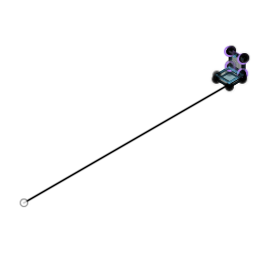
poop-bucket-bucket (Autodesk Fusion 360 design; units mm, degrees)
Autodesk Fusion 360 part; units mm, degrees
sketch "Sketch5" plane through (0, 0, 0) normal (0, 0, 1) x (1, 0, 0)
  line L0 (0, 0) -> (180, 0)
  line L1 (180, 0) -> (180, 80)
  line L2 (180, 80) -> (0, 80)
  line L3 (0, 80) -> (0, 0)
  line L4 (180, 0) -> (130, 0)
  line L5 (130, 0) -> (130, 40)
  line L6 (130, 40) -> (180, 40)
  line L7 (180, 40) -> (180, 0)
  dimension "d5" = 180
  dimension "d6" = 80
  dimension "d7" = 50
  dimension "d8" = 40
  constraint horizontal L0
  constraint vertical L1
  constraint horizontal L2
  constraint vertical L3
  constraint coincident L0.start L3.end
  constraint horizontal L4
  constraint vertical L5
  constraint horizontal L6
  constraint vertical L7
  measures "d5" distance of L0.start L0.end
  measures "d6" distance of L0.start L2.end
  measures "d7" distance of L0.end L4.end
  measures "d8" distance of L0.end L6.end
sketch "Sketch6" plane through (0, 0, 50) normal (0, 0, 1) x (-1, 0, 0)
  line L0 (-130, -40) -> (-180, -40)
  line L1 (-180, -40) -> (-180, -80)
  line L2 (-180, -80) -> (0, -80)
  line L3 (0, -80) -> (0, 0)
  line L4 (0, 0) -> (-130, 0)
  line L5 (-130, 0) -> (-130, -40)
  line L6 (-4, -76) -> (-126, -76)
  line L7 (-126, -76) -> (-126, -4)
  line L8 (-126, -4) -> (-4, -4)
  line L9 (-4, -4) -> (-4, -76)
  line L10 (-126, -76) -> (-176, -76)
  line L11 (-176, -76) -> (-176, -44)
  line L12 (-176, -44) -> (-126, -44)
  line L13 (-126, -44) -> (-126, -76)
  dimension "d11" = 4
  dimension "d12" = 4
  dimension "d13" = 4
  dimension "d14" = 4
  dimension "d15" = 4
  dimension "d16" = 4
  constraint horizontal L6
  constraint vertical L7
  constraint horizontal L8
  constraint vertical L9
  constraint horizontal L10
  constraint vertical L11
  constraint horizontal L12
  constraint vertical L13
  measures "d11" distance of L4 L8
  measures "d12" distance of L3 L9
  measures "d13" distance of L2 L6
  measures "d14" distance of L5 L7
  measures "d15" distance of L0 L12
  measures "d16" distance of L1 L11
sketch "Sketch7" plane through (0, 0, 50) normal (0, 0, 1) x (-1, 0, 0)
  line L0 (-4, -76) -> (-176, -76)
  line L1 (-176, -76) -> (-176, -44)
  line L2 (-176, -44) -> (-126, -44)
  line L3 (-126, -44) -> (-126, -4)
  line L4 (-126, -4) -> (-4, -4)
  line L5 (-4, -4) -> (-4, -76)
  line L6 (-130, -40) -> (-180, -40)
  line L7 (-180, -40) -> (-180, -80)
  line L8 (-180, -80) -> (0, -80)
  line L9 (0, -80) -> (0, 0)
  line L10 (0, 0) -> (-130, 0)
  line L11 (-130, 0) -> (-130, -40)
  line L12 (-4, -76) -> (0, -76)
  line L13 (-176, -44) -> (-176, -40)
  constraint coincident L0.start L5.end
  constraint coincident L9 L12.end
  constraint perpendicular L9 L12
  constraint coincident L1.end L2.start
  constraint coincident L6 L13.end
  constraint perpendicular L6 L13
sketch "Sketch8" plane through (0, 40, 0) normal (0, -1, 0) x (1, 0, 0)
  line L0 (180, 50) -> (180, 110)
  line L1 (180, 110) -> (176, 110)
  line L2 (176, 110) -> (176, 50)
  line L3 (176, 50) -> (180, 50)
  line L4 (176, 50) -> (180, 50)
  constraint coincident L2.end L3.start
  constraint coincident L0 L3.end
  constraint perpendicular L0 L3
sketch "Sketch9" plane through (0, 0, 110) normal (0, 0, 1) x (-1, 0, 0)
  line L0 (-180, -40) -> (-180, -80)
  line L1 (-180, -80) -> (0, -80)
  line L2 (0, -76) -> (-176, -76)
  line L3 (-176, -76) -> (-176, -40)
  line L4 (0, -80) -> (0, -76)
  line L5 (-176, -40) -> (-180, -40)
  line L6 (0, -80) -> (0, -76)
  constraint coincident L1.end L4.start
  constraint coincident L2 L4.end
  constraint perpendicular L2 L4
sketch "Sketch10" plane through (0, 80, 0) normal (0, 1, 0) x (-1, 0, 0)
  spline S0 degree 3 poles (-63.037188, 47.973181) (-57.805899, 55.776696) (-62.188829, 66.234353) (-72.120703, 68.166657) knots 0 0 0 0 1 1 1 1
  spline S1 degree 3 poles (-72.120703, 68.166657) (-66.968789, 73.015993) (-71.009453, 80.172126) (-76.645078, 82.707205) knots 0 0 0 0 1 1 1 1
  spline S2 degree 3 poles (-76.645078, 82.707205) (-79.507501, 83.994509) (-80.596523, 85.515174) (-81.546485, 87.100136) knots 0 0 0 0 1 1 1 1
  spline S3 degree 3 poles (-81.546485, 87.100136) (-83.367188, 90.128768) (-84.036953, 94.472168) (-88.819297, 96.945176) knots 0 0 0 0 1 1 1 1
  spline S4 degree 3 poles (-88.819297, 96.945176) (-92.113359, 98.651738) (-96.771718, 99.105604) (-99.272031, 97.627324) knots 0 0 0 0 1 1 1 1
  spline S5 degree 3 poles (-99.272031, 97.627324) (-100.953827, 96.635137) (-99.00406, 96.178731) (-97.565468, 95.015411) knots 0 0 0 0 1 1 1 1
  spline S6 degree 3 poles (-97.565468, 95.015411) (-95.179296, 93.083106) (-95.065156, 90.017326) (-97.153672, 87.554161) knots 0 0 0 0 1 1 1 1
  spline S7 degree 3 poles (-97.153672, 87.554161) (-99.8375, 84.381701) (-101.995547, 83.617638) (-104.421406, 82.707365) knots 0 0 0 0 1 1 1 1
  spline S8 degree 3 poles (-104.421406, 82.707365) (-110.205939, 80.539475) (-114.189452, 73.016153) (-109.040078, 68.166817) knots 0 0 0 0 1 1 1 1
  spline S9 degree 3 poles (-109.040078, 68.166817) (-119.120703, 66.204827) (-123.416955, 55.456818) (-117.798632, 47.618536) knots 0 0 0 0 1 1 1 1
  spline S10 degree 3 poles (-117.798632, 47.618536) (-124.786015, 45.986422) (-130, 39.730723) (-130, 32.242164) knots 0 0 0 0 1 1 1 1
  spline S11 degree 3 poles (-130, 32.242164) (-130, 27.415211) (-127.82957, 23.101656) (-124.418985, 20.20193) knots 0 0 0 0 1 1 1 1
  line L0 (-124.418985, 20.20193) -> (-54.301016, 20.20193)
  spline S12 degree 3 poles (-54.301016, 20.20193) (-50.892813, 23.101661) (-48.72, 27.415056) (-48.72, 32.242164) knots 0 0 0 0 1 1 1 1
  spline S13 degree 3 poles (-48.72, 32.242164) (-48.72, 40.469859) (-55.005547, 47.221657) (-63.037188, 47.973181) knots 0 0 0 0 1 1 1 1
  line L1 (-180, 50) -> (0, 50)
  line L2 (0, 50) -> (0, 110)
  line L3 (0, 110) -> (-180, 110)
  line L4 (-180, 110) -> (-180, 50)
sketch "Sketch11" plane through (0, 78.1, 0) normal (0, 1, 0) x (-1, 0, 0)
  spline S0 degree 3 poles (-72.120703, 68.166657) (-63.027473, 66.397516) (-58.585649, 57.481991) (-61.915206, 50) knots -1 -1 -1 -1 -0.08443962 -0.08443962 -0.08443962 -0.08443962
  spline S1 degree 3 poles (-76.645078, 82.707205) (-71.009453, 80.172126) (-66.968789, 73.015993) (-72.120703, 68.166657) knots -1 -1 -1 -1 0 0 0 0
  spline S2 degree 3 poles (-81.546485, 87.100136) (-80.596523, 85.515174) (-79.507501, 83.994509) (-76.645078, 82.707205) knots -1 -1 -1 -1 0 0 0 0
  spline S3 degree 3 poles (-88.819297, 96.945176) (-84.036953, 94.472168) (-83.367188, 90.128768) (-81.546485, 87.100136) knots -1 -1 -1 -1 0 0 0 0
  spline S4 degree 3 poles (-99.272031, 97.627324) (-96.771718, 99.105604) (-92.113359, 98.651738) (-88.819297, 96.945176) knots -1 -1 -1 -1 0 0 0 0
  spline S5 degree 3 poles (-97.565468, 95.015411) (-99.00406, 96.178731) (-100.953827, 96.635137) (-99.272031, 97.627324) knots -1 -1 -1 -1 0 0 0 0
  spline S6 degree 3 poles (-97.153672, 87.554161) (-95.065156, 90.017326) (-95.179296, 93.083106) (-97.565468, 95.015411) knots -1 -1 -1 -1 0 0 0 0
  spline S7 degree 3 poles (-104.421406, 82.707365) (-101.995547, 83.617638) (-99.8375, 84.381701) (-97.153672, 87.554161) knots -1 -1 -1 -1 0 0 0 0
  spline S8 degree 3 poles (-109.040078, 68.166817) (-114.189452, 73.016153) (-110.205939, 80.539475) (-104.421406, 82.707365) knots -1 -1 -1 -1 0 0 0 0
  spline S9 degree 3 poles (-119.170519, 50) (-122.517702, 57.482369) (-118.131108, 66.397432) (-109.040078, 68.166817) knots -0.90183199 -0.90183199 -0.90183199 -0.90183199 0 0 0 0
  line L0 (-95.271606, 70.572289) -> (-74.970963, 70.04733) construction
  line L1 (-74.970963, 70.04733) -> (-74.728394, 79.427711) construction
  line L2 (-74.728394, 79.427711) -> (-95.029037, 79.95267) construction
  line L3 (-95.029037, 79.95267) -> (-95.271606, 70.572289) construction
  line L4 (-119.170519, 50) -> (-61.915206, 50)
  dimension "d43" = 10
sketch "Sketch12" plane through (0, 78.1, 0) normal (0, 1, 0) x (-1, 0, 0)
  line L0 (-95.287543, 69.956012) -> (-95.029389, 79.939051)
  line L1 (-95.029389, 79.939051) -> (-93.803641, 79.907354)
  line L2 (-93.803641, 79.907354) -> (-94.061795, 69.924315)
  line L3 (-94.061795, 69.924315) -> (-95.287543, 69.956012)
  spline S0 degree 3 poles (-72.120703, 68.166657) (-63.027473, 66.397516) (-58.585649, 57.481991) (-61.915206, 50) knots -1 -1 -1 -1 -0.08443962 -0.08443962 -0.08443962 -0.08443962
  spline S1 degree 3 poles (-76.645078, 82.707205) (-71.009453, 80.172126) (-66.968789, 73.015993) (-72.120703, 68.166657) knots -1 -1 -1 -1 0 0 0 0
  spline S2 degree 3 poles (-81.546485, 87.100136) (-80.596523, 85.515174) (-79.507501, 83.994509) (-76.645078, 82.707205) knots -1 -1 -1 -1 0 0 0 0
  spline S3 degree 3 poles (-88.819297, 96.945176) (-84.036953, 94.472168) (-83.367188, 90.128768) (-81.546485, 87.100136) knots -1 -1 -1 -1 0 0 0 0
  spline S4 degree 3 poles (-99.272031, 97.627324) (-96.771718, 99.105604) (-92.113359, 98.651738) (-88.819297, 96.945176) knots -1 -1 -1 -1 0 0 0 0
  spline S5 degree 3 poles (-97.565468, 95.015411) (-99.00406, 96.178731) (-100.953827, 96.635137) (-99.272031, 97.627324) knots -1 -1 -1 -1 0 0 0 0
  spline S6 degree 3 poles (-97.153672, 87.554161) (-95.065156, 90.017326) (-95.179296, 93.083106) (-97.565468, 95.015411) knots -1 -1 -1 -1 0 0 0 0
  spline S7 degree 3 poles (-104.421406, 82.707365) (-101.995547, 83.617638) (-99.8375, 84.381701) (-97.153672, 87.554161) knots -1 -1 -1 -1 0 0 0 0
  spline S8 degree 3 poles (-109.040078, 68.166817) (-114.189452, 73.016153) (-110.205939, 80.539475) (-104.421406, 82.707365) knots -1 -1 -1 -1 0 0 0 0
  spline S9 degree 3 poles (-119.170519, 50) (-122.517702, 57.482369) (-118.131108, 66.397432) (-109.040078, 68.166817) knots -0.90183199 -0.90183199 -0.90183199 -0.90183199 0 0 0 0
  line L4 (-87.151, 72.076086) -> (-85.888444, 71.886709)
  spline S10 degree 3 poles (-85.888444, 71.886709) (-86.013749, 71.544143) (-86.256236, 70.881215) (-86.786653, 70.416925) (-87.042978, 70.192555) knots 0 0 0 0 0.10747009 0.20797433 0.20797433 0.20797433 0.20797433
  spline S11 degree 3 poles (-87.042978, 70.192555) (-87.34739, 70.021715) (-87.993643, 69.659028) (-88.736198, 69.642145) (-89.128979, 69.633214) knots 0 0 0 0 0.10312117 0.21892194 0.21892194 0.21892194 0.21892194
  spline S12 degree 3 poles (-89.128979, 69.633214) (-89.621732, 69.678688) (-90.564027, 69.765647) (-91.278869, 70.381614) (-91.619899, 70.675474) knots 0 0 0 0 0.14436887 0.2760774 0.2760774 0.2760774 0.2760774
  spline S13 degree 3 poles (-91.619899, 70.675474) (-91.880847, 71.060122) (-92.4446, 71.891114) (-92.466685, 72.89904) (-92.478547, 73.44042) knots 0 0 0 0 0.13656936 0.29504448 0.29504448 0.29504448 0.29504448
  spline S14 degree 3 poles (-92.478547, 73.44042) (-92.438608, 73.998404) (-92.364473, 75.03413) (-91.749305, 75.865486) (-91.465551, 76.24896) knots 0 0 0 0 0.16381985 0.30408105 0.30408105 0.30408105 0.30408105
  spline S15 degree 3 poles (-91.465551, 76.24896) (-91.115766, 76.534017) (-90.399204, 77.11798) (-89.474783, 77.168101) (-89.001612, 77.193755) knots 0 0 0 0 0.13181373 0.2700304 0.2700304 0.2700304 0.2700304
  spline S16 degree 3 poles (-89.001612, 77.193755) (-88.544529, 77.144258) (-87.648774, 77.047256) (-86.983276, 76.441647) (-86.657366, 76.145067) knots 0 0 0 0 0.13410505 0.26280803 0.26280803 0.26280803 0.26280803
  spline S17 degree 3 poles (-86.657366, 76.145067) (-86.399569, 75.755215) (-85.840301, 74.909463) (-85.820549, 73.891605) (-85.809902, 73.342931) knots 0 0 0 0 0.13742972 0.29814259 0.29814259 0.29814259 0.29814259
  spline S18 degree 3 poles (-85.809902, 73.342931) (-85.811508, 73.297542) (-85.815363, 73.188589) (-85.821553, 73.079742) (-85.825164, 73.016241) knots 0 0 0 0 0.01362508 0.03270546 0.03270546 0.03270546 0.03270546
  line L5 (-85.825164, 73.016241) -> (-91.218456, 73.155707)
  spline S19 degree 3 poles (-91.218456, 73.155707) (-91.192425, 72.791673) (-91.144397, 72.120013) (-90.765174, 71.566695) (-90.591487, 71.313271) knots 0 0 0 0 0.10717868 0.19774945 0.19774945 0.19774945 0.19774945
  spline S20 degree 3 poles (-90.591487, 71.313271) (-90.380387, 71.12298) (-89.95425, 70.738849) (-89.383911, 70.673733) (-89.096108, 70.640875) knots 0 0 0 0 0.08305336 0.16765533 0.16765533 0.16765533 0.16765533
  spline S21 degree 3 poles (-89.096108, 70.640875) (-88.882219, 70.64798) (-88.46859, 70.661722) (-88.109509, 70.866388) (-87.936109, 70.965221) knots 0 0 0 0 0.06312425 0.12207286 0.12207286 0.12207286 0.12207286
  spline S22 degree 3 poles (-87.936109, 70.965221) (-87.778407, 71.106547) (-87.433022, 71.416068) (-87.250294, 71.843706) (-87.151, 72.076086) knots 0 0 0 0 0.06278045 0.13749631 0.13749631 0.13749631 0.13749631
  line L6 (-103.914159, 49.813108) -> (-85.96986, 50.017766) construction
  line L7 (-85.96986, 50.017766) -> (-86.085841, 60.186892) construction
  line L8 (-86.085841, 60.186892) -> (-104.03014, 59.982234) construction
  line L9 (-104.03014, 59.982234) -> (-103.914159, 49.813108) construction
  line L10 (-109.465848, 33.644768) -> (-81.410898, 33.591101) construction
  line L11 (-81.410898, 33.591101) -> (-81.399171, 39.721358) construction
  line L12 (-81.399171, 39.721358) -> (-109.454121, 39.775026) construction
  line L13 (-109.454121, 39.775026) -> (-109.465848, 33.644768) construction
  line L14 (-119.170519, 50) -> (-61.915206, 50)
  dimension "d46" = 10
  dimension "d47" = 10
sketch "Sketch13" plane through (0, 0, 0) normal (0, 0, -1) x (1, 0, 0)
  arc A0 (180, -50) -> (170, -40) centre (170, -50) ccw
  line L0 (170, -40) -> (135, -40)
  arc A1 (130, -35) -> (135, -40) centre (135, -35) ccw
  line L1 (130, -35) -> (130, -10)
  arc A2 (130, -10) -> (120, 0) centre (120, -10) ccw
  line L2 (120, 0) -> (10, 0)
  arc A3 (10, 0) -> (0, -10) centre (10, -10) ccw
  line L3 (0, -10) -> (0, -70)
  arc A4 (0, -70) -> (10, -80) centre (10, -70) ccw
  line L4 (10, -80) -> (170, -80)
  arc A5 (170, -80) -> (180, -70) centre (170, -70) ccw
  line L5 (180, -70) -> (180, -50)
  circle A6 centre (12, -2) radius 1.25
  circle A7 centre (12, -78) radius 1.25
  circle A8 centre (168, -78) radius 1.25
  dimension "d50" = 2.5
  dimension "d51" = 12
  dimension "d52" = 2
  dimension "d53" = 2.5
  dimension "d54" = 2
  dimension "d55" = 12
  dimension "d56" = 2.5
  dimension "d57" = 12
  dimension "d58" = 2
  measures "d50" diameter of A6
  measures "d51" distance of L3 A6.centre
  measures "d52" distance of L2 A6.centre
  measures "d53" diameter of A7
  measures "d54" distance of L4 A7.centre
  measures "d55" distance of L3 A7.centre
  measures "d56" diameter of A8
  measures "d57" distance of L5 A8.centre
  measures "d58" distance of L4 A8.centre
sketch "Sketch14" plane through (0, 0, 0) normal (0, -1, 0) x (1, 0, 0)
  line L0 (120, 47) -> (10, 47)
  line L1 (10, 47) -> (10, 0)
  line L2 (10, 0) -> (120, 0)
  line L3 (120, 0) -> (120, 47)
  line L4 (0, 25) -> (176, 25)
  line L5 (176, 25) -> (176, 56.725104)
  line L6 (176, 56.725104) -> (0, 56.725104)
  line L7 (0, 56.725104) -> (0, 25)
  dimension "d65" = 176
  constraint horizontal L4
  constraint vertical L5
  constraint horizontal L6
  constraint vertical L7
  measures "d65" distance of L4.start L4.end
sketch "Sketch15" plane through (0, 40, 0) normal (0, -1, 0) x (1, 0, 0)
  line L0 (176.000003, 25) -> (135.000002, 0)
  line L1 (135.000002, 0) -> (176.000003, 0)
  line L2 (176.000003, 0) -> (176.000003, 25)
  constraint horizontal L1
  constraint perpendicular L1 L2
sketch "Sketch16" plane through (0, 0, 4) normal (0, 0, 1) x (-1, 0, 0)
  arc A0 (-171, -44) -> (-176, -49) centre (-171, -49) ccw
  line L0 (-176, -49) -> (-176, -76)
  line L1 (-176, -76) -> (-9, -76)
  arc A1 (-9, -76) -> (-4, -71) centre (-9, -71) ccw
  line L2 (-4, -71) -> (-4, -9)
  arc A2 (-4, -9) -> (-9, -4) centre (-9, -9) ccw
  line L3 (-9, -4) -> (-121, -4)
  arc A3 (-121, -4) -> (-126, -9) centre (-121, -9) ccw
  line L4 (-126, -9) -> (-126, -39)
  arc A4 (-131, -44) -> (-126, -39) centre (-131, -39) ccw
  line L5 (-131, -44) -> (-171, -44)
  line L6 (-141.561257, -76.000004) -> (-141.561257, -44)
  constraint perpendicular L5 L6
sketch "Sketch17" plane through (0, 0, 4) normal (0, 0, 1) x (-1, 0, 0)
  arc A0 (-171, -44) -> (-176, -49) centre (-171, -49) ccw
  line L0 (-176, -49) -> (-176, -76)
  line L1 (-176, -76) -> (-9, -76)
  arc A1 (-9, -76) -> (-4, -71) centre (-9, -71) ccw
  line L2 (-4, -71) -> (-4, -9)
  arc A2 (-4, -9) -> (-9, -4) centre (-9, -9) ccw
  line L3 (-9, -4) -> (-121, -4)
  arc A3 (-121, -4) -> (-126, -9) centre (-121, -9) ccw
  line L4 (-126, -9) -> (-126, -39)
  arc A4 (-131, -44) -> (-126, -39) centre (-131, -39) ccw
  line L5 (-131, -44) -> (-171, -44)
sketch "Sketch18" plane through (0, 0, 0) normal (0, 0, 1) x (1, 0, 0)
  line L0 (250, 0) -> (430, 0)
  line L1 (430, 0) -> (430, 180)
  line L2 (430, 180) -> (250, 180)
  line L3 (250, 180) -> (250, 0)
  dimension "d76" = 180
  dimension "d77" = 180
  constraint horizontal L0
  constraint vertical L1
  constraint horizontal L2
  constraint vertical L3
  measures "d76" distance of L0.start L0.end
  measures "d77" distance of L0.start L2.end
extrude "Extrude12" add sketch "Sketch18" along normal blind 4 makes body 1
sketch "Sketch19" plane through (0, 0, 4) normal (0, 0, 1) x (-1, 0, 0)
  line L0 (-250, -180) -> (-250, 0)
  line L1 (-250, 0) -> (-430, 0)
  line L2 (-430, 0) -> (-430, -180)
  line L3 (-430, -180) -> (-250, -180)
  line L4 (-258, -8) -> (-422, -8)
  line L5 (-422, -8) -> (-422, -172)
  line L6 (-422, -172) -> (-258, -172)
  line L7 (-258, -172) -> (-258, -8)
  dimension "d80" = 164
  dimension "d81" = 164
  dimension "d82" = 8
  dimension "d83" = 8
  constraint horizontal L4
  constraint vertical L5
  constraint horizontal L6
  constraint vertical L7
  measures "d80" distance of L4.start L4.end
  measures "d81" distance of L4.start L6.end
  measures "d82" distance of L1 L4
  measures "d83" distance of L0 L7
extrude "Extrude13" add sketch "Sketch19" along normal blind 2 bodies 1
sketch "Sketch20" plane through (0, 0, 6) normal (0, 0, 1) x (-1, 0, 0)
  line L0 (-258, -8) -> (-258, -172)
  line L1 (-258, -172) -> (-422, -172)
  line L2 (-422, -172) -> (-422, -8)
  line L3 (-422, -8) -> (-258, -8)
  line L4 (-430, -180) -> (-250, -180)
  line L5 (-250, -180) -> (-250, 0)
  line L6 (-250, 0) -> (-430, 0)
  line L7 (-430, 0) -> (-430, -180)
  line L8 (-256, -174) -> (-424, -174)
  line L9 (-424, -174) -> (-424, -6)
  line L10 (-424, -6) -> (-256, -6)
  line L11 (-256, -6) -> (-256, -174)
  dimension "d86" = 168
  dimension "d87" = 168
  dimension "d88" = 6
  dimension "d89" = 6
  constraint horizontal L8
  constraint vertical L9
  constraint horizontal L10
  constraint vertical L11
  measures "d86" distance of L8.start L8.end
  measures "d87" distance of L8.start L10.end
  measures "d88" distance of L4 L8
  measures "d89" distance of L5 L11
extrude "Extrude14" add sketch "Sketch20" along normal blind 50 contours L8 L9 L10 L11 picked at (-367.333333, -6.666667) bodies 1
sketch "Sketch21" plane through (0, 0, 6) normal (0, 0, 1) x (-1, 0, 0)
  line L0 (-256, -6) -> (-256, -174)
  line L1 (-256, -174) -> (-424, -174)
  line L2 (-424, -174) -> (-424, -6)
  line L3 (-424, -6) -> (-256, -6)
  line L4 (-430, -180) -> (-250, -180)
  line L5 (-250, -180) -> (-250, 0)
  line L6 (-250, 0) -> (-430, 0)
  line L7 (-430, 0) -> (-430, -180)
  line L8 (-250, 0) -> (-256, 0)
  line L9 (-256, 0) -> (-256, -6)
  line L10 (-256, -6) -> (-250, -6)
  line L11 (-250, -6) -> (-250, 0)
  line L12 (-424, -6) -> (-430, -6)
  line L13 (-430, -6) -> (-430, 0)
  line L14 (-430, 0) -> (-424, 0)
  line L15 (-424, 0) -> (-424, -6)
  line L16 (-424, -174) -> (-430, -174)
  line L17 (-430, -174) -> (-430, -180)
  line L18 (-430, -180) -> (-424, -180)
  line L19 (-424, -180) -> (-424, -174)
  line L20 (-250, -180) -> (-256, -180)
  line L21 (-256, -180) -> (-256, -174)
  line L22 (-256, -174) -> (-250, -174)
  line L23 (-250, -174) -> (-250, -180)
  constraint horizontal L8
  constraint vertical L9
  constraint horizontal L10
  constraint vertical L11
  constraint coincident L0.start L3.end
  constraint coincident L5.end L6.start
  constraint horizontal L12
  constraint vertical L13
  constraint horizontal L14
  constraint vertical L15
  constraint coincident L6.end L7.start
  constraint coincident L2.end L3.start
  constraint horizontal L16
  constraint vertical L17
  constraint horizontal L18
  constraint vertical L19
  constraint coincident L4.start L7.end
  constraint coincident L1.end L2.start
  constraint horizontal L20
  constraint vertical L21
  constraint horizontal L22
  constraint vertical L23
  constraint coincident L0.end L1.start
  constraint coincident L4.end L5.start
extrude "Extrude15" add sketch "Sketch21" along normal blind 50 separate body contours L4 L5 L20 L21 L22 L23 picked at (-254, -176) makes body 2
extrude "Extrude16" add sketch "Sketch21" along normal blind 50 separate body contours L5 L6 L8 L9 L10 L11 picked at (-254, -4) makes body 3
extrude "Extrude17" add sketch "Sketch21" along normal blind 50 separate body contours L6 L7 L12 L13 L14 L15 picked at (-426, -4) makes body 4
extrude "Extrude18" add sketch "Sketch21" along normal blind 50 separate body contours L4 L7 L16 L17 L18 L19 picked at (-428, -178) makes body 5
sketch "Sketch22" plane through (0, 0, 56) normal (0, 0, 1) x (-1, 0, 0)
  line L0 (-250, -6) -> (-250, 0)
  line L1 (-250, 0) -> (-256, 0)
  line L2 (-256, 0) -> (-256, -6)
  line L3 (-256, -6) -> (-250, -6)
  line L4 (-250, -180) -> (-430, -180)
  line L5 (-430, -180) -> (-430, 0)
  line L6 (-430, 0) -> (-250, 0)
  line L7 (-250, 0) -> (-250, -180)
  line L8 (-256, -6) -> (-424.000006, -6)
  line L9 (-424.000006, -6) -> (-424.000006, -174.000003)
  line L10 (-424.000006, -174.000003) -> (-256, -174.000003)
  line L11 (-256, -174.000003) -> (-256, -6)
  constraint horizontal L4
  constraint vertical L5
  constraint horizontal L6
  constraint vertical L7
  constraint horizontal L8
  constraint vertical L9
  constraint horizontal L10
  constraint vertical L11
  constraint coincident L2.end L3.start
extrude "Extrude19" add sketch "Sketch22" along normal blind 6 separate body contours L2 L3 L4 L5 L6 L7 picked at (-312, -178.000001) makes body 6
extrude "Extrude20" add 1 faces at (254, 4, 56) along direction (0, 0, 1) blind 6 on bodies 3 bodies 1 2 4 5 3 6
sketch "Sketch23" plane through (0, 0, 62) normal (0, 0, 1) x (-1, 0, 0)
  line L0 (-256, -6) -> (-256, -174.000003)
  line L1 (-256, -174.000003) -> (-424.000006, -174.000003)
  line L2 (-424.000006, -174.000003) -> (-424.000006, -6)
  line L3 (-424.000006, -6) -> (-256, -6)
  line L4 (-250, -180) -> (-250, 0)
  line L5 (-250, 0) -> (-430, 0)
  line L6 (-430, 0) -> (-430, -180)
  line L7 (-430, -180) -> (-250, -180)
  line L8 (-250, -180) -> (-430, -180)
  line L9 (-430, -180) -> (-430, -186)
  line L10 (-430, -186) -> (-250, -186)
  line L11 (-250, -186) -> (-250, -180)
  line L12 (-250, -180) -> (-256, -180)
  line L13 (-256, -180) -> (-256, -210)
  line L14 (-256, -210) -> (-250, -210)
  line L15 (-250, -210) -> (-250, -180)
  line L16 (-250, -210) -> (-430, -210)
  line L17 (-430, -210) -> (-430, -204)
  line L18 (-430, -204) -> (-250, -204)
  line L19 (-250, -204) -> (-250, -210)
  line L20 (-430, -210) -> (-424, -210)
  line L21 (-424, -210) -> (-424, -180)
  line L22 (-424, -180) -> (-430, -180)
  line L23 (-430, -180) -> (-430, -210)
  dimension "d104" = 180
  dimension "d105" = 6
  dimension "d106" = 6
  dimension "d107" = 30
  dimension "d108" = 180
  dimension "d109" = 6
  dimension "d110" = 6
  dimension "d111" = 30
  constraint horizontal L8
  constraint vertical L9
  constraint horizontal L10
  constraint vertical L11
  constraint coincident L4.start L7.end
  constraint horizontal L12
  constraint vertical L13
  constraint horizontal L14
  constraint vertical L15
  constraint horizontal L16
  constraint vertical L17
  constraint horizontal L18
  constraint vertical L19
  constraint horizontal L20
  constraint vertical L21
  constraint horizontal L22
  constraint vertical L23
  measures "d104" distance of L4.start L6.end
  measures "d105" distance of L4.start L10.end
  measures "d106" distance of L4.start L12.end
  measures "d107" distance of L4.start L14.end
  measures "d108" distance of L14.end L16.end
  measures "d109" distance of L14.end L18.end
  measures "d110" distance of L16.end L20.end
  measures "d111" distance of L16.end L6.end
extrude "Extrude21" add sketch "Sketch23" along normal blind 6 separate body contours L7 L8 L10 L11 L12 L13 L15 | L7 L8 L10 L13 L21 | L10 L13 L15 L18 | L7 L8 L9 L10 L21 L22 L23 | L10 L13 L18 L21 | L13 L14 L15 L16 L18 L19 | L10 L18 L21 L23 | L13 L16 L18 L21 | L16 L17 L18 L20 L21 L23 picked at (-254, -184) picked at (-368, -182) picked at (-254, -192) picked at (-428, -184) picked at (-368, -198) picked at (-254, -208) picked at (-428, -192) picked at (-368, -206) picked at (-428, -208) makes body 7
extrude "Extrude22" add sketch "Sketch23" along normal blind 180 separate body contours L10 L13 L18 L21 picked at (-368, -198) makes body 8
extrude "Extrude23" add sketch "Sketch23" along normal blind 180 separate body contours L7 L8 L10 L11 L12 L13 L15 | L7 L8 L9 L10 L21 L22 L23 | L13 L14 L15 L16 L18 L19 | L16 L17 L18 L20 L21 L23 picked at (-254, -184) picked at (-428, -184) picked at (-254, -208) picked at (-428, -208) makes body 9 at (424, 184, 122) makes body 10 at (250, 208, 122) makes body 11 at (424, 208, 122) makes body 12 at (250, 184, 122)
extrude "Extrude24" cut 1 faces at (368, 198, 242) along direction (0, 0, -1) blind 6 on bodies 8 bodies 8
extrude "Extrude25" cut sketch "Sketch23" along normal blind 6 contours L10 L13 L18 L21 picked at (-368, -198) bodies 8
sketch "Sketch24" plane through (256, 0, 0) normal (1, 0, 0) x (0, 1, 0)
  line L0 (204, 62) -> (210, 62)
  line L1 (210, 62) -> (210, 242)
  line L2 (210, 242) -> (204, 242)
  line L3 (204, 242) -> (204, 62)
  line L4 (186.000003, 68.000001) -> (180.000003, 68.000001)
  line L5 (180.000003, 68.000001) -> (180.000003, 62.000001)
  line L6 (180.000003, 62.000001) -> (186.000003, 62.000001)
  line L7 (186.000003, 62.000001) -> (186.000003, 68.000001)
  line L8 (204, 62) -> (210.000003, 62)
  line L9 (210.000003, 62) -> (210.000003, 68.000001)
  line L10 (210.000003, 68.000001) -> (204, 68.000001)
  line L11 (204, 68.000001) -> (204, 62)
  constraint horizontal L4
  constraint vertical L5
  constraint horizontal L6
  constraint vertical L7
  constraint horizontal L8
  constraint vertical L9
  constraint horizontal L10
  constraint vertical L11
  constraint coincident L0.start L3.end
extrude "Extrude26" add sketch "Sketch24" along normal blind 168 contours L0 L1 L3 L8 L9 L10 L11 picked at (206, 66.000001) bodies 8 9 12 10 11
extrude "Extrude27" add sketch "Sketch24" along normal blind 168 contours L4 L5 L6 L7 picked at (182.000003, 66.000001) bodies 1 2 4 5 9 8 12
sketch "Sketch25" plane through (0, 186, 0) normal (0, 1, 0) x (-1, 0, 0)
  line L0 (-256, 62) -> (-250, 62)
  line L1 (-250, 62) -> (-250, 242)
  line L2 (-250, 242) -> (-256, 242)
  line L3 (-256, 242) -> (-256, 236)
  line L4 (-256, 236) -> (-256, 68)
  line L5 (-256, 68) -> (-424, 68)
  line L6 (-424, 68) -> (-424, 236)
  line L7 (-424, 236) -> (-424, 242)
  line L8 (-424, 242) -> (-430, 242)
  line L9 (-430, 242) -> (-430, 62)
  line L10 (-430, 62) -> (-424, 62)
  line L11 (-424, 62) -> (-256, 62)
  line L12 (-256, 62) -> (-250.000004, 62)
  line L13 (-250.000004, 62) -> (-250.000004, 68.000001)
  line L14 (-250.000004, 68.000001) -> (-256, 68.000001)
  line L15 (-256, 68.000001) -> (-256, 62)
  line L16 (-430, 62) -> (-424, 62)
  line L17 (-424, 62) -> (-424, 68)
  line L18 (-424, 68) -> (-430, 68)
  line L19 (-430, 68) -> (-430, 62)
  constraint horizontal L12
  constraint vertical L13
  constraint horizontal L14
  constraint vertical L15
  constraint coincident L0.start L11.end
  constraint horizontal L16
  constraint vertical L17
  constraint horizontal L18
  constraint vertical L19
  constraint coincident L5.end L6.start
  constraint coincident L9.end L10.start
extrude "Extrude28" add sketch "Sketch25" along normal blind 18 separate body contours L9 L10 L16 L17 L18 L19 picked at (-426, 64) makes body 13
extrude "Extrude29" add sketch "Sketch25" along normal blind 18 separate body contours L0 L1 L12 L13 L14 L15 picked at (-254, 64) makes body 14
sketch "Sketch26" plane through (424, 0, 0) normal (-1, 0, 0) x (0, -1, 0)
  line L0 (-210.000003, 68.000001) -> (-204, 68)
  line L1 (-204, 68) -> (-204, 236)
  line L2 (-204, 236) -> (-204, 242)
  line L3 (-204, 242) -> (-210, 242)
  line L4 (-210, 242) -> (-210.000003, 68.000001)
  line L5 (-210, 242) -> (-204, 242)
  line L6 (-204, 242) -> (-204, 236)
  line L7 (-204, 236) -> (-210, 236)
  line L8 (-210, 236) -> (-210, 242)
  line L9 (-186.000003, 242.000004) -> (-180.000003, 242.000004)
  line L10 (-180.000003, 242.000004) -> (-180.000003, 236.000004)
  line L11 (-180.000003, 236.000004) -> (-186.000003, 236.000004)
  line L12 (-186.000003, 236.000004) -> (-186.000003, 242.000004)
  constraint horizontal L5
  constraint vertical L6
  constraint horizontal L7
  constraint vertical L8
  constraint coincident L1.end L2.start
  constraint coincident L3.end L4.start
  constraint horizontal L9
  constraint vertical L10
  constraint horizontal L11
  constraint vertical L12
sketch "Sketch27" plane through (0, 204, 0) normal (0, -1, 0) x (1, 0, 0)
  line L0 (250, 62) -> (430, 62)
  line L1 (430, 62) -> (430, 242)
  line L2 (430, 242) -> (424, 242)
  line L3 (424, 242) -> (424, 236)
  line L4 (424, 236) -> (424, 68)
  line L5 (424, 68) -> (256, 68)
  line L6 (256, 68) -> (256, 236)
  line L7 (256, 236) -> (256, 242)
  line L8 (256, 242) -> (250, 242)
  line L9 (250, 242) -> (250, 62)
  line L10 (250, 242) -> (256, 242)
  line L11 (256, 242) -> (256, 236)
  line L12 (256, 236) -> (250, 236)
  line L13 (250, 236) -> (250, 242)
  line L14 (424, 242) -> (430, 242)
  line L15 (430, 242) -> (430, 236)
  line L16 (430, 236) -> (424, 236)
  line L17 (424, 236) -> (424, 242)
  constraint horizontal L10
  constraint vertical L11
  constraint horizontal L12
  constraint vertical L13
  constraint coincident L6.end L7.start
  constraint coincident L8.end L9.start
  constraint horizontal L14
  constraint vertical L15
  constraint horizontal L16
  constraint vertical L17
  constraint coincident L1 L15.end
  constraint coincident L2.end L3.start
extrude "Extrude30" add sketch "Sketch26" along normal blind 168 separate body contours L2 L3 L4 L5 L6 L7 L8 picked at (-208, 238) makes body 15
extrude "Extrude31" add sketch "Sketch26" along normal blind 168 separate body contours L9 L10 L11 L12 picked at (-184.000003, 240.000004) makes body 16
extrude "Extrude32" add sketch "Sketch27" along normal blind 18 separate body contours L1 L2 L3 L14 L15 L16 L17 picked at (428, 238) makes body 17
extrude "Extrude33" add sketch "Sketch27" along normal blind 18 separate body contours L7 L8 L9 L10 L11 L12 L13 picked at (252, 238) makes body 18
sketch "Sketch28" plane through (0, 0, 242.000004) normal (0, 0, 1) x (-1, 0, 0)
  line L0 (-424, -180.000003) -> (-424, -186.000003)
  line L1 (-424, -186.000003) -> (-256, -186.000003)
  line L2 (-256, -186.000003) -> (-256, -180.000003)
  line L3 (-256, -180.000003) -> (-424, -180.000003)
  line L4 (-330, -190) -> (-350, -190)
  line L5 (-350, -190) -> (-350, -155)
  line L6 (-350, -155) -> (-330, -155)
  line L7 (-330, -155) -> (-330, -190)
  line L8 (-335, -185) -> (-345, -185)
  line L9 (-345, -185) -> (-345, -160)
  line L10 (-345, -160) -> (-335, -160)
  line L11 (-335, -160) -> (-335, -185)
  line L12 (-250, -210) -> (-250, -180)
  line L13 (-430, -180) -> (-430, -210)
  line L14 (-250, -210) -> (-430, -210)
  dimension "d138" = 80
  dimension "d139" = 85
  dimension "d140" = 80
  dimension "d141" = 20
  dimension "d142" = 25
  constraint horizontal L4
  constraint vertical L5
  constraint horizontal L6
  constraint vertical L7
  constraint horizontal L8
  constraint vertical L9
  constraint horizontal L10
  constraint vertical L11
  measures "d138" distance of L7 L12
  measures "d139" distance of L9 L13
  measures "d140" distance of L5 L13
  measures "d141" distance of L4 L14
  measures "d142" distance of L8 L14
extrude "Extrude34" add sketch "Sketch28" along normal blind 10 contours L3 L5 L6 L7 L9 L10 L11 | L1 L3 L5 L7 L8 L9 L11 | L1 L4 L5 L7 picked at (-348.333333, -165.000001) picked at (-348.333333, -183.666668) picked at (-343.333333, -187.333335) bodies 16
extrude "Extrude35" add 1 faces at (343.333333, 187.333335, 242.000004) along direction (0, 0, -1) blind 6 on bodies 16 bodies 16
sketch "Sketch29" plane through (0, 186, 0) normal (0, -1, 0) x (1, 0, 0)
  line L0 (256, 68) -> (424, 68)
  line L1 (424, 68) -> (424, 236)
  line L2 (424, 236) -> (256, 236)
  line L3 (256, 236) -> (256, 68)
  line L4 (258, 70) -> (422, 70)
  line L5 (422, 70) -> (422, 234)
  line L6 (422, 234) -> (258, 234)
  line L7 (258, 234) -> (258, 70)
  line L8 (256, 68) -> (424, 68)
  line L9 (422, 234) -> (424.000006, 234)
  line L10 (258, 234) -> (256.000004, 234)
  dimension "d147" = 164
  dimension "d148" = 164
  dimension "d149" = 2
  dimension "d150" = 2
  constraint horizontal L4
  constraint vertical L5
  constraint horizontal L6
  constraint vertical L7
  constraint perpendicular L1 L9
  constraint perpendicular L3 L10
  measures "d147" distance of L4.start L4.end
  measures "d148" distance of L4.start L6.end
  measures "d149" distance of L4 L8
  measures "d150" distance of L3 L7
extrude "Extrude36" cut sketch "Sketch29" against normal blind 16 contours L4 L5 L6 L7 picked at (312.666667, 179.333333) bodies 1
sketch "Sketch30" plane through (258, 0, 0) normal (1, 0, 0) x (0, 1, 0)
  line L0 (186, 234) -> (186, 70)
  line L1 (186, 70) -> (202, 70)
  line L2 (202, 70) -> (202, 234)
  line L3 (202, 234) -> (186, 234)
  arc A0 (186, 70) -> (202, 85.999989) centre (180.000003, 92.000001) ccw
  constraint coincident L0.end L1.start
sketch "Sketch31" plane through (430, 0, 0) normal (1, 0, 0) x (0, 1, 0)
  line L0 (180, 62) -> (210, 62)
  line L1 (210, 62) -> (210, 68)
  line L2 (210, 68) -> (180, 68)
  line L3 (180, 68) -> (180, 62)
  arc A0 (210, 62.000001) -> (180.000003, 32) centre (210.000003, 32) ccw
  arc A1 (210.000003, 62.000001) -> (180.000003, 32) centre (210.000003, 32) ccw
  line L4 (180.000003, 32) -> (180, 62)
  constraint coincident L0.end L1.start
  constraint coincident L0.start L3.end
sketch "Sketch32" plane through (430, 0, 0) normal (1, 0, 0) x (0, 1, 0)
  line L0 (186, 68) -> (186, 62)
  line L1 (186, 62) -> (204, 62)
  line L2 (204, 62) -> (204, 68)
  line L3 (204, 68) -> (186, 68)
sketch "Sketch33" plane through (430, 0, 0) normal (1, 0, 0) x (0, 1, 0)
extrude "Extrude37" add sketch "Sketch31" against normal blind 180 contours L0 A0 A1 L4 picked at (185.893898, 56.106103) bodies 1 4 15 16 17 18 2 5 7 13 14
sketch "Sketch34" plane through (424, 0, 0) normal (-1, 0, 0) x (0, -1, 0)
  line L0 (-180, 6) -> (-174, 6)
  line L1 (-174, 6) -> (-174, 56)
  line L2 (-174, 56) -> (-180, 56)
  line L3 (-180, 56) -> (-180.000003, 32)
  line L4 (-180.000003, 32) -> (-180, 6)
  line L5 (-180.000003, 32) -> (-174, 32)
  line L6 (-180.000003, 32) -> (2768.758397, 32.000305)
  constraint coincident L1 L5.end
  constraint perpendicular L1 L5
  constraint perpendicular L4 L6
extrude "Extrude38" add sketch "Sketch21" along normal blind 30 separate body contours L1 L4 L19 L21 picked at (-312, -178) makes body 19
sketch "Sketch35" plane through (0, 0, 0) normal (0, 0, 1) x (1, 0, 0)
  line L0 (260, 10) -> (420, 10)
  line L1 (420, 10) -> (420, 170)
  line L2 (420, 170) -> (260, 170)
  line L3 (260, 170) -> (260, 10)
  line L4 (250, 0) -> (430, 0)
  line L5 (250, 180) -> (250, 0)
  circle A0 centre (417.5, 30) radius 1
  circle A1 centre (417.5, 150) radius 1
  circle A2 centre (262.5, 150) radius 1
  circle A3 centre (262.5, 30) radius 1
  dimension "d157" = 160
  dimension "d158" = 160
  dimension "d159" = 10
  dimension "d160" = 10
  dimension "d161" = 2
  dimension "d162" = 20
  dimension "d163" = 2.5
  dimension "d164" = 2
  dimension "d165" = 20
  dimension "d166" = 2.5
  dimension "d167" = 2
  dimension "d168" = 2.5
  dimension "d169" = 20
  dimension "d170" = 2
  dimension "d171" = 20
  dimension "d172" = 2.5
  constraint horizontal L0
  constraint vertical L1
  constraint horizontal L2
  constraint vertical L3
  measures "d157" distance of L0.start L0.end
  measures "d158" distance of L0.start L2.end
  measures "d159" distance of L0 L4
  measures "d160" distance of L3 L5
  measures "d161" diameter of A0
  measures "d162" distance of L0 A0.centre
  measures "d163" distance of L1 A0.centre
  measures "d164" diameter of A1
  measures "d165" distance of L2 A1.centre
  measures "d166" distance of L1 A1.centre
  measures "d167" diameter of A2
  measures "d168" distance of L3 A2.centre
  measures "d169" distance of L2 A2.centre
  measures "d170" diameter of A3
  measures "d171" distance of L0 A3.centre
  measures "d172" distance of L3 A3.centre
extrude "Extrude39" add sketch "Sketch35" against normal blind 10 separate body contours A0 | A1 | A2 | A3 picked at (416.891254, 29.812227) picked at (417.574174, 149.675024) picked at (262.574174, 149.675024) picked at (261.891254, 29.812227) makes body 20 at (262.624344, 30.992239, -6.666667) makes body 21 at (417.624344, 30.992239, -6.666667) makes body 22 at (262.624344, 150.992239, -6.666667) makes body 23 at (417.624344, 150.992239, -6.666667)
fillet "Fillet16" radius 1 4 edges at (261.567673, 30.361615, -10) (416.567673, 30.361615, -10) (261.567673, 150.361615, -10) (416.567673, 150.361615, -10) on bodies 20 21 22 23
sketch "Sketch36" plane through (430, 0, 0) normal (1, 0, 0) x (0, 1, 0)
  line L0 (210, 62) -> (210, 242)
  line L1 (210, 242) -> (204, 242)
  line L2 (204, 242) -> (204, 68)
  line L3 (204, 68) -> (186, 68)
  line L4 (186, 68) -> (186, 242)
  line L5 (186, 242) -> (180, 242)
  line L6 (180, 242) -> (180, 62)
  line L7 (180, 62) -> (0, 62)
  line L8 (0, 62) -> (0, 56)
  line L9 (0, 56) -> (174, 56)
  line L10 (174, 56) -> (174, 6)
  line L11 (174, 6) -> (0, 6)
  line L12 (0, 6) -> (0, 0)
  line L13 (0, 0) -> (180, 0)
  line L14 (180, 0) -> (180, 32)
  arc A0 (210, 62) -> (180.000004, 32) centre (210.000003, 32) ccw
  arc A1 (174.000003, 62.000001) -> (180.000003, 68.000001) centre (174.000003, 68.000001) ccw
extrude "Extrude40" add sketch "Sketch36" against normal blind 180 separate body contours L6 L7 A1 picked at (178.821222, 63.17878) makes body 24
sketch "Sketch37" plane through (0, 186, 0) normal (0, -1, 0) x (1, 0, 0)
  line L0 (258.000004, 234.000003) -> (256.000004, 234.000003)
  line L1 (422.000006, 234.000003) -> (424.000006, 234.000003)
  constraint horizontal L0
  constraint horizontal L1
move_body "Move1" bodies 16 to x (1, 0, 0) y (0, 1, 0) z (0, 0, 1) at (200, 0, 0)
extrude "Extrude41" add sketch "Sketch29" along normal blind 4 separate body contours L1 L2 L3 L6 L9 L10 picked at (367.333333, 235.333333) makes body 25
move_body "Move2" bodies 16 to x (1, 0, 0) y (0, 1, 0) z (0, 0, 1) at (-200, 0, 0)
